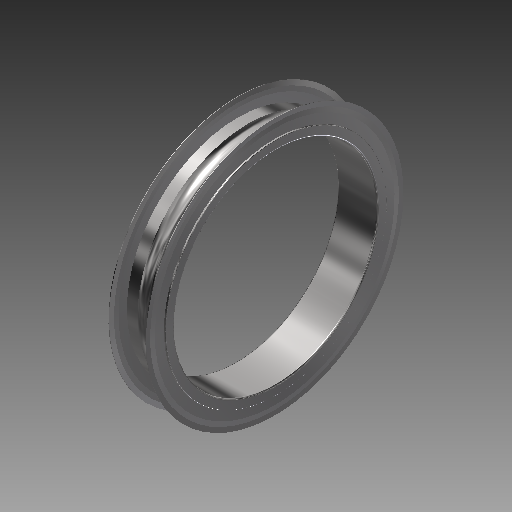
# Autodesk Inventor part: 61807-2RS1_PART1
Saved by Autodesk Inventor 2018 (Build 220112000, 112)
## iProperties
Category: PARTsolutions
Company: SKF
Created: 2019-11-07
Part Number: 61807-2RS1_PART1
Material: Stainless Steel
Catalog Web Link: www.cadenas.de
Description: -Deep groove ball bearings
Vendor: SKF
Document SubType Name: Modeling
Designer: psadmin
Manufacturer: SKF
Mass: 10.1122 g
Surface Area: 35.8838 cm^2
Volume: 1.26402 cm^3
Density: 8 g/cm^3
Appearance: Semi-Polished
PSOL_IDENT_0: {$CADENAS_DATA\23d-libs\skf\bearings_units_and_housings\ball_bearings\deep_groove_ball_bearings\bb1_
PSOL_IDENT_1: 001_101.prj},198 {VTYP=3D},{NB=61807-2RS1_PART1},{LINA=61807-2RS1_PART1},{NN=BB1_001_101_PART1},{NOP
PSOL_IDENT_2: RJ=TRUE},{DATE=07.11.2019 10:38:24},{GEOMDATE=11.06.2019 11:24:58},{VERSION=},{LINEID=7650},{WBVAR=}
PSOL_IDENT_3: ,{WBNUMERIC=}  {NB=61807-2RS1_PART1},{LINA=61807-2RS1_PART1},{KT=DUMMY},{PRODUCTID=1010281807},{DESI
PSOL_IDENT_4: GNATION=61807-2RS1},{DD=35.00},{D=47.000},{B=7.000},{C=0.000},{DD1=38.21},{DD2=0.0},{D1=0.00},{D2=44
PSOL_IDENT_5: .40},{D3=0.00},{D4=0.000},{HH=MIN},{BB=0.000},{FF=0.00},{R0MAX=MIN},{R0=MIN},{R12=0.30},{PITCH=40.50
PSOL_IDENT_6: },{DW=3.500},{DDAMIN=37.000},{DDAMAX=38.000},{DDBMIN=MIN},{DDBMAX=MIN},{DBMIN=MIN},{DAMAX=45.000},{B
PSOL_IDENT_7: BAMIN=MIN},{CAMAX=MIN},{RAMAX=0.300},{LOAD1=4.360},{LOAD2=3.350},{LOAD3=0.140},{SPEED1=MIN},{SPEED2=
PSOL_IDENT_8: 8500},{KR=0.015},{F0=14.300},{Z=19},{II=1},{MASS=0.022},{BEARING=61807-2RS1},{RING=},{HELP=2.078},{H
PSOL_IDENT_9: ELP2=1.300},{DD1ALG=19.105},{YALG=19.105},{PITCH1=40.500},{DW1=3.500},{YALG1=21.422},{HALG1=2.078},{
PSOL_IDENT_10: SH=19.105},{CU=0.700},{DESIGN=dgbb2rs},{HALG=1.605},{B1=0},{ALGO=1.000}
NT: Deep groove ball bearings
NB: 61807-2RS1_PART1
NBSYN: $DESIGNATION._PART1
LINA: 61807-2RS1_PART1
SUPPLIER: SKF
ARTICLENO: 61807-2RS1_PART1
BOMINFO: 61807-2RS1_PART1
CREATOR: CADENAS GmbH
Title: 61807-2RS1_PART1
Author: Cadenas PARTsolutions
Comments: Deep groove ball bearings
Autodesk Inventor part; units mm, degrees
ref_plane "YZ Plane" through (0, 0, 0) normal (1, 0, 0) x (0, 1, 0)
ref_plane "XZ Plane" through (0, 0, 0) normal (0, 1, 0) x (-1, 0, 0)
ref_plane "XY Plane" through (0, 0, 0) normal (0, 0, 1) x (1, 0, 0)
sketch "Sketch_58" plane through (0, 0, 0) normal (0, 0, 1) x (1, 0, 0)
  line L0 (50, 0) -> (-50, 0)
  line L1 (0, 19.005) -> (0, 17.8)
  arc A0 (0, 17.8) -> (0.3, 17.5) centre (0.3, 17.8) ccw
  line L2 (0.3, 17.5) -> (6.7, 17.5)
  arc A1 (6.7, 17.5) -> (7, 17.8) centre (6.7, 17.8) ccw
  line L3 (7, 17.8) -> (7, 19.005)
  arc A2 (7, 19.005) -> (6.9, 19.105) centre (6.9, 19.005) ccw
  line L4 (6.9, 19.105) -> (4.8234, 19.105)
  arc A3 (2.1766, 19.105) -> (4.8234, 19.105) centre (3.5, 20.25) ccw
  line L5 (2.1766, 19.105) -> (0.1, 19.105)
  arc A4 (0.1, 19.105) -> (0, 19.005) centre (0.1, 19.005) ccw
  constraints: 12 end point, 10 point on circle, 5 centre point
revolve "Revolution1" add sketch "Sketch_58" angle 360 about axis through (50, 0, 0) along (1, 0, 0)
sketch "Sketch_60" plane through (0, 0, 0) normal (0, 0, 1) x (1, 0, 0)
  line L0 (50, 0) -> (-50, 0)
  line L1 (0.27, 22.2) -> (0.315, 21.4263)
  line L2 (0.315, 21.4263) -> (0.27, 20.6525)
  line L3 (0.27, 20.6525) -> (0.27, 19.105)
  line L4 (0.27, 19.105) -> (0.36, 19.105)
  line L5 (0.36, 19.105) -> (0.45, 20.6525)
  line L6 (0.45, 20.6525) -> (0.45, 21.4263)
  line L7 (0.45, 21.4263) -> (0.36, 22.2)
  line L8 (0.36, 22.2) -> (0.27, 22.2)
  constraints: 18 end point
revolve "Revolution2" add sketch "Sketch_60" angle 360 about axis through (50, 0, 0) along (1, 0, 0)
sketch "Sketch_61" plane through (0, 0, 0) normal (0, 0, 1) x (1, 0, 0)
  line L0 (50, 0) -> (-50, 0)
  line L1 (6.55, 20.6525) -> (6.64, 19.105)
  line L2 (6.64, 19.105) -> (6.73, 19.105)
  line L3 (6.73, 19.105) -> (6.73, 20.6525)
  line L4 (6.73, 20.6525) -> (6.685, 21.4263)
  line L5 (6.685, 21.4263) -> (6.73, 22.2)
  line L6 (6.73, 22.2) -> (6.64, 22.2)
  line L7 (6.64, 22.2) -> (6.55, 21.4263)
  line L8 (6.55, 21.4263) -> (6.55, 20.6525)
  constraints: 18 end point
revolve "Revolution3" add sketch "Sketch_61" angle 360 about axis through (50, 0, 0) along (1, 0, 0)
body "Solid1"
